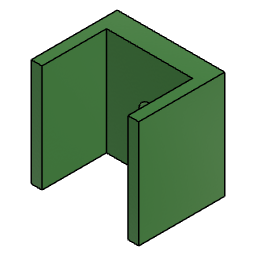
gripper (Autodesk Fusion 360 design; units mm, degrees)
Autodesk Fusion 360 part; units mm, degrees
sketch "Sketch1" plane through (0, 0, 0) normal (0, 1, 0) x (1, 0, 0)
  line L0 (0, 0) -> (100, 0)
  line L1 (100, 0) -> (100, -100)
  line L2 (100, -100) -> (0, -100)
  line L3 (0, -100) -> (0, 0)
  dimension "d1" = 100
  dimension "d2" = 100
  constraint horizontal L0
  constraint vertical L1
  constraint horizontal L2
  constraint vertical L3
  constraint coincident L0.start L3.end
  measures "d1" distance of L0.start L0.end
  measures "d2" distance of L0.start L2.end
extrude "Extrude1" add sketch "Sketch1" along normal blind 20
sketch "Sketch2" plane through (0, 0, 0) normal (0, -1, 0) x (1, 0, 0)
  line L0 (100, 100) -> (0, 100)
  line L1 (0, 100) -> (0, 0)
  line L2 (0, 0) -> (100, 0)
  line L3 (100, 0) -> (100, 100)
  line L4 (10, 100) -> (90, 100)
  line L5 (90, 100) -> (90, 0)
  line L6 (90, 0) -> (10, 0)
  line L7 (10, 0) -> (10, 100)
  dimension "d5" = 10
  dimension "d6" = 80
  constraint horizontal L4
  constraint vertical L5
  constraint horizontal L6
  constraint vertical L7
  constraint coincident L2 L5.end
  constraint coincident L0 L4.start
  measures "d5" distance of L3 L5
  measures "d6" distance of L4.start L4.end
extrude "Extrude2" add sketch "Sketch2" along normal blind 60 contours L0 L2 L3 L5 | L0 L1 L2 L7
sketch "Sketch3" plane through (0, 0, 0) normal (0, -1, 0) x (1, 0, 0)
  line L0 (10, 100) -> (10, 0)
  line L1 (10, 0) -> (90, 0)
  line L2 (90, 0) -> (90, 100)
  line L3 (90, 100) -> (10, 100)
  circle A0 centre (50, 50) radius 10
  dimension "d9" = 20
  measures "d9" diameter of A0
extrude "Extrude3" cut sketch "Sketch3" against normal blind 20 contours A0
scale "Scale1" factor 2.5 about (0, 0, 0) bodies 1
